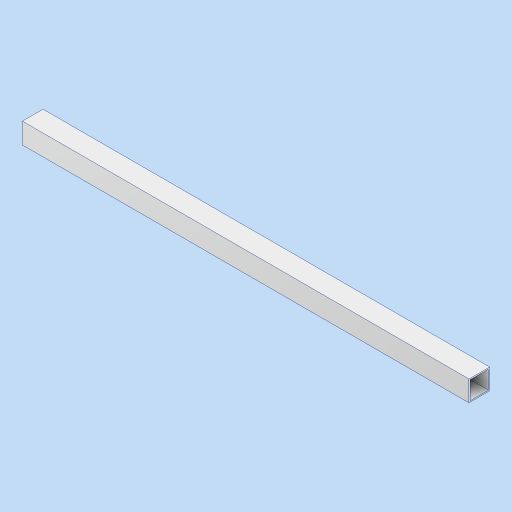
# Autodesk Inventor part: 44.92cmTube
Saved by Autodesk Inventor 2024 (Build 280153000, 153)
## iProperties
Created: 2023-10-19
Part Number: 44.92cmTube
Material: Aluminum 6061
Document SubType Name: Modeling
Designer: megan
Density: 2.7 g/cm^3
Appearance: Aluminum - Flat
Author: megan
Autodesk Inventor part; units mm, degrees
ref_plane "YZ Plane" through (0, 0, 0) normal (1, 0, 0) x (0, 1, 0)
ref_plane "XZ Plane" through (0, 0, 0) normal (0, 1, 0) x (-1, 0, 0)
ref_plane "XY Plane" through (0, 0, 0) normal (0, 0, 1) x (1, 0, 0)
sketch "Sketch1" plane through (0, 0, 0) normal (1, 0, 0) x (0, 1, 0)
  line L0 (0, 0) -> (-25.4, 0)
  line L1 (-25.4, 0) -> (-25.4, -25.4)
  line L2 (-25.4, -25.4) -> (0, -25.4)
  line L3 (0, -25.4) -> (0, 0)
  line L4 (-1.5875, -23.8125) -> (-23.8125, -23.8125)
  line L5 (-23.8125, -23.8125) -> (-23.8125, -1.5875)
  line L6 (-23.8125, -1.5875) -> (-1.5875, -1.5875)
  line L7 (-1.5875, -1.5875) -> (-1.5875, -23.8125)
  point P0 (-12.7, -23.8125)
  point P1 (-12.7, -25.4)
  point P2 (-23.8125, -12.7)
  point P3 (-1.5875, -12.7)
  dimension "d0" = 25.4
  dimension "d1" = 25.4
  dimension "d2" = 1.5875
  dimension "d3" = 1.5875
  dimension "d4" = 1.5875
  dimension "d5" = 1.5875
  constraints: 16 end point, 4 midpoint, 4 parallel, 2 horizontal, 2 perpendicular
  measures "d0" distance of L2.end L1.end
  measures "d1" distance of L1.end L0.end
  measures "d2" distance of point (-12.7, -23.812) point (-12.7, -25.4)
  measures "d3" distance from line of L1 point (-23.812, -12.7)
  measures "d4" distance from line of L3 point (-1.587, -12.7)
  measures "d5" distance between parallel lines of L0 L6
extrude "Extrusion1" add sketch "Sketch1" along normal blind 549.2
body "Solid1"
